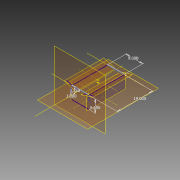
# Autodesk Inventor part: Wheelbase
Saved by Autodesk Inventor 2015 (Build 190159000, 159)
## iProperties
Created: 2016-01-19
Part Number: Wheelbase
Material: Generic
Document SubType Name: Modeling
Designer: sethbattis
Density: 1 g/cm^3
Appearance: Default
Author: sethbattis
Autodesk Inventor part; units mm, degrees
ref_plane "YZ Plane" through (0, 0, 0) normal (1, 0, 0) x (0, 1, 0)
sketch "Dimensions" plane through (0, 0, 0) normal (0, 1, 0) x (-1, 0, 0)
  line L0 (262.3048, 0) -> (-262.3048, 0) construction
  line L1 (0, -337.82) -> (0, 337.82) construction
  line L2 (114.3, 241.3) -> (114.3, -241.3) construction
  line L3 (-114.3, 241.3) -> (-114.3, -241.3) construction
  line L4 (114.3, -241.3) -> (-114.3, -241.3) construction
  line L5 (114.3, 241.3) -> (-114.3, 241.3) construction
  point P0 (0, 0)
  dimension "d61" = 228.6
  dimension "d62" = 482.6
  constraints: 8 coincident, 8 end point, 2 vertical, 1 horizontal, 1 perpendicular, 2 other
  measures "d61" distance of L4.start L4.end
  measures "d62" distance of L3.start L3.end
ref_plane "Kingpin Vertical Plane End C" through (-114.3, 0, 241.3) normal (0, 0, 1) x (1, 0, 0)
sketch "Kingpin Angles" plane through (-114.3, 0, 241.3) normal (0, 0, 1) x (1, 0, 0)
  line L0 (-73.0606, 22.4802) -> (73.0606, -22.4802)
  line L1 (301.6606, 22.4802) -> (155.5394, -22.4802)
  line L2 (0, -169.0624) -> (228.6, -169.0624)
  line L3 (0, 0) -> (-25.4, -82.55) construction
  line L4 (-25.4, -82.55) -> (0, -82.55) construction
  line L5 (0, -82.55) -> (0, 0) construction
  line L6 (228.6, 0) -> (254, -82.55) construction
  line L7 (254, -82.55) -> (228.6, -82.55) construction
  line L8 (228.6, -82.55) -> (228.6, 0) construction
  point P0 (114.3, 0)
  dimension "d67" = 169.0624
  dimension "d70" = 25.4
  dimension "d71" = 82.55
  constraints: 18 end point, 4 perpendicular, 3 equal length, 3 horizontal, 2 midpoint
  measures "d67" distance from line of L2 L6.start
  measures "d70" distance of L3.end L4.end
  measures "d71" distance of L4.end L3.start
ref_plane "Kingpin Tops Side A" through (-187.3606, 22.4802, 241.3) normal (0.2940858, 0.955779, 0) x (0.955779, -0.2940858, 0)
ref_plane "Kingpin Tops Side B" through (41.2394, -22.4802, 241.3) normal (-0.2940858, 0.955779, 0) x (0.955779, 0.2940858, 0)
sketch "Sketch15" plane through (-187.3606, 22.4802, 241.3) normal (0.2940858, 0.955779, 0) x (0.955779, -0.2940858, 0)
  line L0 (76.4409, 0) -> (76.4409, 482.6)
  point P0 (185.6864, 241.3)
  constraints: 2 end point, 1 vertical
sketch "Sketch16" plane through (41.2394, -22.4802, 241.3) normal (-0.2940858, 0.955779, 0) x (0.955779, 0.2940858, 0)
  line L0 (76.4409, 0) -> (76.4409, 482.6)
  point P0 (-32.8047, 241.3)
  constraints: 2 end point, 1 vertical
ref_plane "Ground Plane (Dead Ahead)" through (-114.3, -169.0624, 241.3) normal (0, 1, 0) x (1, 0, 0)
sketch "Ground Center" plane through (-114.3, -169.0624, 241.3) normal (0, 1, 0) x (1, 0, 0)
  line L0 (114.3, 579.12) -> (114.3, -96.52) construction
  line L1 (-148.0048, 241.3) -> (376.6048, 241.3) construction
  point P0 (114.3, 241.3)
  point P1 (114.3, 241.3)
  constraints: 1 coincident
ref_plane "Axle Ends" through (114.3, 0, 241.3) normal (-1, 0, 0) x (0, 0, -1)
sketch "Sketch18" plane through (114.3, 0, 241.3) normal (-1, 0, 0) x (0, 0, -1)
  circle A0 centre (0, 0) radius 9.525
  circle A1 centre (484.4419, 0) radius 9.525
  point P0 (241.3, 0)
  dimension "d73" = 19.05
  dimension "d74" = 19.05
  constraints: 2 centre point
  measures "d73" diameter of A0
  measures "d74" diameter of A1
extrude "Axles" add sketch "Sketch18" along normal up to surface (228.6 mm away)
body "Solid6"
